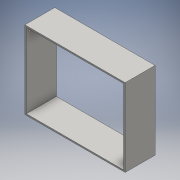
# Autodesk Inventor part: veggur
Saved by Autodesk Inventor 2016 (Build 200138000, 138)
## iProperties
Created: 2016-02-20
Part Number: veggur
Material: Generic
Document SubType Name: Modeling
Designer: Róbert
Density: 1 g/cm^3
Appearance: Default
Author: Róbert
Autodesk Inventor part; units mm, degrees
ref_plane "YZ Plane" through (0, 0, 0) normal (1, 0, 0) x (0, 1, 0)
ref_plane "XZ Plane" through (0, 0, 0) normal (0, 1, 0) x (-1, 0, 0)
ref_plane "XY Plane" through (0, 0, 0) normal (0, 0, 1) x (1, 0, 0)
sketch "Sketch1" plane through (0, 0, 0) normal (0, 1, 0) x (-1, 0, 0)
  line L0 (0, 0) -> (0, -50)
  line L1 (0, -50) -> (-65, -50)
  line L2 (-65, -50) -> (-65, 0)
  line L3 (-65, 0) -> (0, 0)
  line L4 (-66, -51) -> (1, -51)
  line L5 (1, -51) -> (1, 1)
  line L6 (1, 1) -> (-66, 1)
  line L7 (-66, 1) -> (-66, -51)
  dimension "d0" = 50
  dimension "d1" = 65
  dimension "d2" = 1
  constraints: 16 end point, 4 perpendicular, 2 vertical, 3 other
  measures "d0" distance of L0.start L0.end
  measures "d1" distance of L0.end L1.end
  measures "d2" distance between parallel lines of L1 L4
extrude "Extrusion1" add sketch "Sketch1" along normal blind 20
sketch "Sketch2" plane through (-1, 0, -51) normal (-1, 0, 0) x (0, 0, 1)
  line L0 (0, 0) -> (0, 20) projected
  line L1 (0, 10) -> (52, 10)
  line L2 (52, 0) -> (52, 20) projected
  line L3 (0, 0) -> (52, 0)
  line L4 (51, 0) -> (1, 0) projected
  point P0 (48, 2.138)
  constraints: 4 end point, 2 midpoint, 1 collinear
hole "Hole1" at (-1, 2.138, -3) direction (1, 0, 0) diameter 1.2 depth 8 tip angle 118
body "Solid1"
